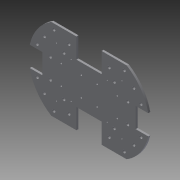
# Autodesk Inventor part: base
Saved by Autodesk Inventor 2015 (Build 190159000, 159)
## iProperties
Created: 2014-09-21
Part Number: base
Material: Générique
Document SubType Name: Modeling
Designer: astralien3000
Density: 1 g/cm^3
Appearance: Par défaut
Author: astralien3000
Autodesk Inventor part; units mm, degrees
ref_plane "YZ Plane" through (0, 0, 0) normal (1, 0, 0) x (0, 1, 0)
ref_plane "XZ Plane" through (0, 0, 0) normal (0, 1, 0) x (-1, 0, 0)
ref_plane "XY Plane" through (0, 0, 0) normal (0, 0, 1) x (1, 0, 0)
sketch "Esquisse1" plane through (0, 0, 0) normal (0, 1, 0) x (-1, 0, 0)
  circle A0 centre (0, 0) radius 25 construction
  line L0 (-25, 0) -> (25, 0) construction
  arc A1 (-75, -80.7775) -> (-75, 80.7775) centre (-25, 0) ccw construction
  arc A2 (75, 80.7775) -> (75, -80.7775) centre (25, 0) ccw construction
  line L1 (0, 25) -> (0, 0) construction
  line L2 (-75, 80.7775) -> (75, 80.7775)
  line L3 (-75, -80.7775) -> (75, -80.7775)
  arc A3 (75, -80.7775) -> (75, 80.7775) centre (25, 0) ccw
  arc A4 (-75, 80.7775) -> (-75, -80.7775) centre (-25, 0) ccw
  dimension "d0" = 50
  dimension "d1" = 190
  dimension "d2" = 150
  constraints: 11 point on circle, 8 end point, 5 centre point, 3 coincident, 2 perpendicular, 1 horizontal, 1 midpoint, 2 other
  measures "d0" diameter of A0
  measures "d1" diameter of A1
  measures "d2" distance of L2.start L2.end
extrude "Extrusion1" add sketch "Esquisse1" along normal blind 4
sketch "Esquisse4" plane through (0, 0, 0) normal (0, -1, 0) x (1, 0, 0)
  line L0 (-50, 40) -> (50, 40) construction
  line L1 (50, 40) -> (50, -40) construction
  line L2 (50, -40) -> (-50, -40) construction
  line L3 (-50, -40) -> (-50, 40) construction
  circle A0 centre (-50, 40) radius 3
  circle A1 centre (50, 40) radius 3
  circle A2 centre (50, -40) radius 3
  circle A3 centre (-50, -40) radius 3
  line L4 (75, 80.7775) -> (-75, 80.7775) projected
  point P0 (0, 0)
  dimension "d15" = 80
  dimension "d16" = 100
  dimension "d17" = 50
  dimension "d18" = 40
  dimension "d19" = 6
  dimension "d20" = 6
  dimension "d21" = 6
  dimension "d22" = 6
  dimension "d25" = 40.7775
  constraints: 8 end point, 4 centre point, 4 coincident, 2 parallel, 1 horizontal, 1 perpendicular
  measures "d15" distance of L0.end L1.end
  measures "d16" distance of L0.start L0.end
  measures "d17" distance from line of L1 point (0, 0)
  measures "d18" distance from line of L2 point (0, 0)
  measures "d19" diameter of A0
  measures "d20" diameter of A1
  measures "d21" diameter of A2
  measures "d22" diameter of A3
  measures "d25" distance between parallel lines of L4 L0
extrude "Extrusion4" cut sketch "Esquisse4" against normal through all
sketch "Esquisse8" plane through (0, 0, 0) normal (0, -1, 0) x (1, 0, 0)
  line L0 (96.5, 35) -> (96.5, -35) projected
  line L1 (82, 42) -> (96, 42)
  line L2 (96, 42) -> (96, -42)
  line L3 (96, -42) -> (82, -42)
  line L4 (82, -42) -> (82, 42)
  line L5 (96, 21.5) -> (108.5, 21.5)
  line L6 (108.5, 21.5) -> (108.5, -21.5)
  line L7 (108.5, -21.5) -> (96, -21.5)
  line L8 (96, -21.5) -> (96, 21.5)
  line L9 (82, -14.7) -> (76.3, -14.7)
  line L10 (76.3, -14.7) -> (76.3, 14.7)
  line L11 (76.3, 14.7) -> (82, 14.7)
  line L12 (82, 14.7) -> (82, -14.7)
  line L13 (82, 14.7) -> (72, 14.7)
  line L14 (72, 14.7) -> (72, 24.7)
  line L15 (72, 24.7) -> (82, 24.7)
  line L16 (82, 24.7) -> (82, 14.7)
  line L17 (96, 21.5) -> (110.5, 21.5)
  line L18 (110.5, 21.5) -> (110.5, 35.5)
  line L19 (110.5, 35.5) -> (96, 35.5)
  line L20 (96, 35.5) -> (96, 21.5)
  line L21 (96, 42) -> (82, 42)
  line L22 (82, 42) -> (82, 56)
  line L23 (82, 56) -> (96, 56)
  line L24 (96, 56) -> (96, 42)
  line L25 (72, 24.7) -> (82, 14.7) construction
  line L26 (82, 24.7) -> (72, 14.7) construction
  line L27 (110.5, 21.5) -> (96, 35.5) construction
  line L28 (96, 21.5) -> (110.5, 35.5) construction
  line L29 (82, 56) -> (96, 42) construction
  line L30 (82, 42) -> (96, 56) construction
  circle A0 centre (89, 49) radius 3
  circle A1 centre (77, 19.7) radius 3
  circle A2 centre (103.25, 28.5) radius 3
  arc A3 (75, -80.7775) -> (75, 80.7775) centre (25, 0) ccw projected
  line L31 (108.5, 21.5) -> (115, 21.5)
  line L32 (115, 21.5) -> (115, -21.5)
  line L33 (115, -21.5) -> (108.5, -21.5)
  line L34 (108.5, -21.5) -> (108.5, 21.5)
  line L35 (0, 0) -> (120, 0)
  dimension "d59" = 84
  dimension "d60" = 14
  dimension "d61" = 29.4
  dimension "d62" = 5.7
  dimension "d63" = 12.5
  dimension "d64" = 43
  dimension "d65" = 42
  dimension "d66" = 14.7
  dimension "d67" = 21.5
  dimension "d68" = 14
  dimension "d69" = 14
  dimension "d70" = 14
  dimension "d71" = 10
  dimension "d72" = 10
  dimension "d73" = 6
  dimension "d74" = 6
  dimension "d75" = 6
  dimension "d78" = 6.5
  dimension "d79" = 5
  constraints: 70 end point, 14 parallel, 8 perpendicular, 7 horizontal, 3 centre point, 3 midpoint, 3 point on line, 2 collinear, 1 point on circle
  measures "d59" distance of L3.end L1.start
  measures "d60" distance of L1.start L1.end
  measures "d61" distance of L9.end L10.end
  measures "d62" distance of L10.end L11.end
  measures "d63" distance of L5.start L5.end
  measures "d64" distance of L5.end L6.end
  measures "d65" distance from line of L35.start L1
  measures "d66" distance from line of L35.start L11
  measures "d67" distance from line of L35.start L5
  measures "d68" distance between parallel lines of L1 L23
  measures "d69" distance between parallel lines of L0 L18
  measures "d70" distance of L17.end L18.end
  measures "d71" distance between parallel lines of L13 L15
  measures "d72" distance of L14.end L15.end
  measures "d73" diameter of A1
  measures "d74" diameter of A0
  measures "d75" diameter of A2
  measures "d78" distance between parallel lines of L6 L32
  measures "d79" distance from line of L32 L35.end
extrude "Extrusion6" cut sketch "Esquisse8" against normal through all contours A0 | A1 | A2
mirror "Symétrie2" about plane through (0, 0, 0) normal (0, 0, 1) of "Extrusion6"
mirror "Symétrie3" about plane through (0, 0, 0) normal (1, 0, 0) of "Extrusion6", "Symétrie2"
sketch "Esquisse11" plane through (0, 4, 0) normal (0, 1, 0) x (1, 0, 0)
  line L0 (15.75, 19.5) -> (55.75, 19.5)
  line L1 (55.75, 19.5) -> (55.75, -19.5)
  line L2 (55.75, -19.5) -> (15.75, -19.5)
  line L3 (15.75, -19.5) -> (15.75, 19.5)
  line L4 (11.75, 23.5) -> (59.75, 23.5)
  line L5 (59.75, 23.5) -> (59.75, -23.5)
  line L6 (59.75, -23.5) -> (11.75, -23.5)
  line L7 (11.75, -23.5) -> (11.75, 23.5)
  point P0 (0, 0)
  dimension "d103" = 40
  dimension "d104" = 48
  dimension "d105" = 4
  dimension "d106" = 47
  dimension "d107" = 39
  dimension "d108" = 4
  dimension "d109" = 23.5
  dimension "d110" = 11.75
  constraints: 16 end point, 4 parallel, 2 horizontal, 2 perpendicular
  measures "d103" distance between parallel lines of L3 L1
  measures "d104" distance between parallel lines of L7 L5
  measures "d105" distance between parallel lines of L5 L1
  measures "d106" distance between parallel lines of L4 L6
  measures "d107" distance between parallel lines of L2 L0
  measures "d108" distance between parallel lines of L6 L2
  measures "d109" distance from line of point (0, 0) L4
  measures "d110" distance from line of point (0, 0) L7
hole "Perçage1" at (15.75, 4, -19.5) at (55.75, 4, -19.5) at (55.75, 4, 19.5) at (15.75, 4, 19.5) direction (0, -1, 0) diameter 4 end through all
mirror "Symétrie7" about plane through (0, 0, 0) normal (1, 0, 0) of "Perçage1"
sketch "Esquisse12" plane through (0, 4, 0) normal (0, 1, 0) x (1, 0, 0)
  arc A0 (75, -80.7775) -> (75, 80.7775) centre (25, 0) ccw projected
  line L0 (92.8709, 20) -> (117.8709, 20)
  line L1 (117.8709, 20) -> (117.8709, -20)
  line L2 (117.8709, -20) -> (92.8709, -20)
  line L3 (92.8709, -20) -> (92.8709, 20)
  arc A1 (117.8709, 20) -> (117.8709, -20) centre (25, 0) ccw
  arc A2 (117.8709, -20) -> (117.8709, 20) centre (25, 0) ccw
  point P0 (0, 0)
  dimension "d111" = 25
  dimension "d112" = 40
  constraints: 8 end point, 6 point on circle, 2 centre point, 2 parallel, 1 coincident, 1 concentric, 1 horizontal, 1 perpendicular
  measures "d111" distance between parallel lines of L1 L3
  measures "d112" distance between parallel lines of L0 L2
extrude "Extrusion9" cut sketch "Esquisse12" against normal through all contours L1 A0 | L2 L3 L0 L1
mirror "Symétrie8" about plane through (0, 0, 0) normal (1, 0, 0) of "Extrusion9"
sketch "Esquisse14" plane through (0, 0, 0) normal (0, -1, 0) x (1, 0, 0)
  line L0 (75, 80.7775) -> (-75, 80.7775) projected
  line L1 (-25, 80.7775) -> (25, 80.7775)
  line L2 (25, 80.7775) -> (25, 40.7775)
  line L3 (25, 40.7775) -> (-25, 40.7775)
  line L4 (-25, 40.7775) -> (-25, 80.7775)
  point P0 (0, 0)
  dimension "d131" = 50
  dimension "d132" = 25
  dimension "d133" = 40
  constraints: 8 end point, 2 parallel, 1 horizontal, 1 perpendicular, 1 point on line
  measures "d131" distance between parallel lines of L2 L4
  measures "d132" distance from line of point (0, 0) L2
  measures "d133" distance of L3.end L1.start
extrude "Extrusion11" cut sketch "Esquisse14" against normal through all
mirror "Symétrie10" about plane through (0, 0, 0) normal (0, 0, 1) of "Extrusion11"
sketch "Esquisse15" plane through (0, 0, 0) normal (0, -1, 0) x (1, 0, 0)
  line L0 (-40, 60) -> (40, 60) construction
  line L1 (40, 60) -> (40, -60) construction
  line L2 (40, -60) -> (-40, -60) construction
  line L3 (-40, -60) -> (-40, 60) construction
  circle A0 centre (40, 60) radius 3
  circle A1 centre (-40, 60) radius 3
  circle A2 centre (-40, -60) radius 3
  circle A3 centre (40, -60) radius 3
  point P0 (0, 0)
  dimension "d136" = 120
  dimension "d137" = 80
  dimension "d138" = 40
  dimension "d139" = 60
  dimension "d140" = 6
  dimension "d141" = 6
  dimension "d142" = 6
  dimension "d143" = 6
  constraints: 8 end point, 4 centre point, 4 coincident, 2 parallel, 1 horizontal, 1 perpendicular
  measures "d136" distance of L0.end L1.end
  measures "d137" distance of L0.start L0.end
  measures "d138" distance from line of L1 point (0, 0)
  measures "d139" distance from line of point (0, 0) L0
  measures "d140" diameter of A1
  measures "d141" diameter of A0
  measures "d142" diameter of A3
  measures "d143" diameter of A2
extrude "Extrusion12" cut sketch "Esquisse15" against normal through all
sketch "Esquisse16" plane through (0, 0, 0) normal (0, -1, 0) x (1, 0, 0)
  line L0 (-70, 70) -> (70, 70) construction
  line L1 (70, 70) -> (70, -70) construction
  line L2 (70, -70) -> (-70, -70) construction
  line L3 (-70, -70) -> (-70, 70) construction
  circle A0 centre (70, 70) radius 3
  circle A1 centre (-70, 70) radius 3
  circle A2 centre (-70, -70) radius 3
  circle A3 centre (70, -70) radius 3
  point P0 (0, 0)
  dimension "d146" = 140
  dimension "d147" = 140
  dimension "d148" = 6
  dimension "d149" = 6
  dimension "d150" = 6
  dimension "d151" = 6
  dimension "d152" = 70
  dimension "d153" = 70
  constraints: 8 end point, 4 centre point, 4 coincident, 2 parallel, 1 horizontal, 1 perpendicular
  measures "d146" distance between parallel lines of L3 L1
  measures "d147" distance of L0.end L1.end
  measures "d148" diameter of A1
  measures "d149" diameter of A0
  measures "d150" diameter of A3
  measures "d151" diameter of A2
  measures "d152" distance from line of point (0, 0) L1
  measures "d153" distance from line of point (0, 0) L0
extrude "Extrusion13" cut sketch "Esquisse16" against normal through all
sketch "Esquisse17" plane through (0, 0, 0) normal (0, -1, 0) x (1, 0, 0)
  line L0 (-36, 36) -> (36, 36) construction
  line L1 (36, 36) -> (36, -36) construction
  line L2 (36, -36) -> (-36, -36) construction
  line L3 (-36, -36) -> (-36, 36) construction
  circle A0 centre (-36, 36) radius 1.5
  circle A1 centre (36, 36) radius 1.5
  circle A2 centre (36, -36) radius 1.5
  circle A3 centre (-36, -36) radius 1.5
  point P0 (0, 0)
  dimension "d156" = 72
  dimension "d157" = 72
  dimension "d158" = 3
  dimension "d159" = 3
  dimension "d160" = 3
  dimension "d161" = 3
  dimension "d162" = 36
  dimension "d163" = 36
  constraints: 8 end point, 4 centre point, 4 coincident, 2 parallel, 1 horizontal, 1 perpendicular
  measures "d156" distance of L0.end L1.end
  measures "d157" distance of L0.start L0.end
  measures "d158" diameter of A0
  measures "d159" diameter of A1
  measures "d160" diameter of A2
  measures "d161" diameter of A3
  measures "d162" distance from line of point (0, 0) L1
  measures "d163" distance from line of L2 point (0, 0)
extrude "Extrusion14" cut sketch "Esquisse17" against normal through all
sketch "Esquisse18" plane through (0, 0, 0) normal (0, -1, 0) x (1, 0, 0)
  line L0 (-65, 50) -> (65, 50) construction
  line L1 (65, 50) -> (65, -50) construction
  line L2 (65, -50) -> (-65, -50) construction
  line L3 (-65, -50) -> (-65, 50) construction
  circle A0 centre (-65, 50) radius 1.5
  circle A1 centre (65, 50) radius 1.5
  circle A2 centre (65, -50) radius 1.5
  circle A3 centre (-65, -50) radius 1.5
  point P0 (0, 0)
  dimension "d166" = 3
  dimension "d167" = 3
  dimension "d168" = 3
  dimension "d169" = 3
  dimension "d170" = 100
  dimension "d171" = 130
  dimension "d172" = 65
  dimension "d173" = 50
  constraints: 8 end point, 4 centre point, 4 coincident, 2 parallel, 1 horizontal, 1 perpendicular
  measures "d166" diameter of A0
  measures "d167" diameter of A1
  measures "d168" diameter of A3
  measures "d169" diameter of A2
  measures "d170" distance of L0.end L1.end
  measures "d171" distance of L1.end L2.end
  measures "d172" distance from line of L1 point (0, 0)
  measures "d173" distance from line of point (0, 0) L0
extrude "Extrusion15" cut sketch "Esquisse18" against normal through all
equation "\"d17\" = 0.5 * d16"
equation "\"d18\" = 0.5 * d15"
equation "\"d20\" = d19"
equation "\"d21\" = d19"
equation "\"d22\" = d19"
equation "\"d65\" = 0.5 * d59"
equation "\"d66\" = 0.5 * d61"
equation "\"d67\" = 0.5 * d64"
equation "\"d68\" = d60"
equation "\"d70\" = d69"
